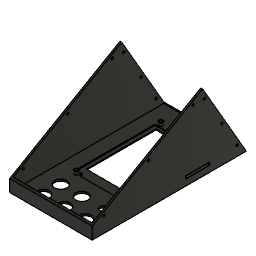
TheShutterTester3_5_screen (Autodesk Fusion 360 design; units mm, degrees)
Autodesk Fusion 360 part; units mm, degrees
sketch "Sketch1" plane through (0, 0, 0) normal (0, 0, 1) x (1, 0, 0)
  line L0 (45, 145.5) -> (45, 50) construction
  line L1 (45, 50) -> (45, 0) construction
  line L2 (0, 14.5) -> (90, 14.5) construction
  line L3 (0, 33.75) -> (90, 33.75) construction
  line L4 (45, 33.75) -> (45, 14.5) construction
  line L5 (22, 33.75) -> (22, 14.5) construction
  line L6 (68, 33.75) -> (68, 14.5) construction
  line L7 (0, 0) -> (90, 0)
  line L8 (90, 0) -> (90, 168)
  line L9 (90, 168) -> (0, 168)
  line L10 (0, 168) -> (0, 0)
  circle A0 centre (45, 33.75) radius 6.7
  circle A1 centre (68, 14.5) radius 6.7
  circle A2 centre (45, 14.5) radius 6.7
  circle A3 centre (22, 14.5) radius 6.7
  circle A4 centre (22, 33.75) radius 6.7
  circle A5 centre (68, 33.75) radius 3.7
  line L11 (13.5, 52) -> (0, 52) construction
  line L12 (13.5, 79) -> (0, 79) construction
  line L13 (73.17, 49) -> (16.83, 49) construction
  line L14 (16.83, 49) -> (16.83, 147) construction
  line L15 (16.83, 147) -> (73.17, 147) construction
  line L16 (73.17, 147) -> (73.17, 49) construction
  circle A6 centre (20.25, 144.5) radius 1.7
  circle A7 centre (69.75, 144.5) radius 1.7
  circle A8 centre (20.25, 52.5) radius 1.7
  circle A9 centre (69.75, 52.5) radius 1.7
  circle A10 centre (20.25, 144.5) radius 2.4
  circle A11 centre (69.75, 52.5) radius 2.4
  line L17 (73.17, 141.0151) -> (72.7211, 141.0151)
  line L18 (73.17, 141.6) -> (16.83, 141.6)
  line L19 (16.83, 141.6) -> (16.83, 55.4)
  line L20 (73.17, 55.4) -> (73.17, 141.6)
  line L21 (20.83, 138.6) -> (20.83, 63)
  line L22 (69.17, 63) -> (69.17, 138.6)
  line L23 (69.17, 138.6) -> (20.83, 138.6)
  circle A12 centre (20.25, 52.5) radius 2.4
  line L24 (66.2226, 55.4) -> (66.2226, 52)
  line L25 (66.2226, 52) -> (57, 52)
  line L26 (66.2226, 55.4) -> (73.17, 55.4)
  line L27 (57, 52) -> (52, 52)
  line L28 (52, 52) -> (24, 52)
  line L29 (24, 52) -> (24, 55.4)
  line L30 (16.83, 55.4) -> (24, 55.4)
  line L31 (45, 55.4) -> (52, 55.4)
  circle A13 centre (69.75, 144.5) radius 2.4
  line L32 (20.83, 63) -> (69.17, 63)
  point P0 (90, 168)
  point P1 (90, 168)
  point P2 (45, 145.5)
  point P3 (45, 0)
  point P4 (17.42, 149)
  point P5 (72.58, 47)
  point P6 (72.58, 149)
  point P7 (22, 33.75)
  point P8 (22, 14.5)
  point P9 (45, 14.5)
  point P10 (45, 33.75)
  point P11 (68, 33.75)
  point P12 (68, 14.5)
  point P13 (0, 158)
  point P14 (90, 0)
  point P15 (110, -10)
  point P16 (17.42, 47)
  point P17 (72.58, 47)
  point P18 (0, 52)
  point P19 (0, 79)
  point P20 (75.5, 98)
  point P21 (45, 97.75)
  point P22 (16.83, 147)
  point P23 (73.17, 49)
  point P24 (69.75, 144.5)
  point P25 (20.25, 144.5)
  point P26 (69.75, 52.5)
  point P27 (20.25, 52.5)
  dimension "d158" = 168
  dimension "d159" = 90
  dimension "d163" = 13.4
  dimension "d165" = 13.4
  dimension "d166" = 13.4
  dimension "d167" = 13.4
  dimension "d190" = 13.4
  dimension "d191" = 7.4
  dimension "d257" = 3.4
  dimension "d258" = 3.4
  dimension "d259" = 3.4
  dimension "d260" = 3.4
  dimension "d261" = 4.8
  dimension "d264" = 4.8
  dimension "d268" = 4.8
  dimension "d280" = 4.8
  constraint coincident P0 L8.end
  constraint coincident P2 L0.start
  constraint coincident P3 L1.end
  constraint horizontal L2
  constraint horizontal L3
  constraint midpoint L3 P10
  constraint midpoint L2 P9
  constraint perpendicular L2 L4
  constraint coincident P7 L5.start
  constraint coincident P8 L5.end
  constraint coincident P9 L4.end
  constraint coincident P10 L4.start
  constraint coincident P11 L6.start
  constraint coincident P12 L6.end
  constraint coincident P17 P5
  constraint horizontal L7
  constraint vertical L8
  constraint horizontal L9
  constraint vertical L10
  constraint coincident P1 P0
  constraint coincident L7.start L10.end
  constraint coincident P18 L11.end
  constraint coincident P19 L12.end
  constraint midpoint L0 P21
  constraint horizontal L13
  constraint vertical L14
  constraint horizontal L15
  constraint vertical L16
  constraint coincident P22 L14.end
  constraint coincident P23 L13.start
  constraint coincident P25 A6.centre
  constraint coincident P24 A7.centre
  constraint coincident P27 A8.centre
  constraint coincident P26 A9.centre
  constraint concentric A9 A11
  constraint coincident L14 L19.end
  constraint coincident L16 L20.start
  constraint perpendicular L16 L26
  constraint coincident L16 L17.start
  constraint perpendicular L16 L17
  constraint coincident L16 L18.start
  constraint coincident L14 L18.end
  constraint perpendicular L14 L18
  constraint perpendicular L13 L24
  constraint perpendicular L24 L25
  constraint collinear L26 L31
  constraint perpendicular L0 L28
  constraint perpendicular L29 L30
  constraint coincident L0 L31.start
  constraint collinear L30 L31
  measures "d158" distance of P14 P1
  measures "d159" distance of P1 L9.end
  measures "d163" diameter of A0
  measures "d165" diameter of A1
  measures "d166" diameter of A2
  measures "d167" diameter of A3
  measures "d190" diameter of A4
  measures "d191" diameter of A5
  measures "d257" diameter of A6
  measures "d258" diameter of A7
  measures "d259" diameter of A8
  measures "d260" diameter of A9
  measures "d261" diameter of A10
  measures "d264" diameter of A11
  measures "d268" diameter of A12
  measures "d280" diameter of A13
extrude "Extrude24" add sketch "Sketch1" along normal blind 2 contours L7 L8 L9 L10
extrude "Extrude21" add sketch "Sketch1" along normal blind 1 contours L18 L19 L20 L24 L25 L26 L27 L28 L29 L30
extrude "Extrude30" add sketch "Sketch1" along normal blind 5 contours A10 | A11 | A12 | A13
sketch "Sketch40" plane through (0, 0, 2) normal (0, 0, 1) x (-1, 0, 0)
  circle A0 centre (-20.25, -52.5) radius 2.4
  circle A1 centre (-20.25, -144.5) radius 2.4
  circle A2 centre (-69.75, -52.5) radius 2.4
  circle A3 centre (-22, -33.75) radius 6.7
  circle A4 centre (-22, -14.5) radius 6.7
  circle A5 centre (-45, -33.75) radius 6.7
  circle A6 centre (-68, -14.5) radius 6.7
  circle A7 centre (-68, -33.75) radius 3.7
  circle A8 centre (-45, -14.5) radius 6.7
  line L0 (0, -168) -> (0, 0)
  line L1 (0, 0) -> (-90, 0)
  line L2 (-90, 0) -> (-90, -168)
  line L3 (-90, -168) -> (0, -168)
  line L4 (0, 0) -> (-90, 0)
  line L5 (0, -168) -> (0, 0)
  line L6 (-90, 0) -> (-90, -168)
  line L7 (-90, -168) -> (0, -168)
  line L8 (-2, -2) -> (-88, -2)
  line L9 (-88, -2) -> (-88, -166)
  line L10 (-88, -166) -> (-2, -166)
  line L11 (-2, -166) -> (-2, -2)
  circle A9 centre (-69.75, -144.5) radius 2.4
  line L12 (-73.17, -55.4) -> (-66.2226, -55.4)
  line L13 (-66.2226, -55.4) -> (-66.2226, -52)
  line L14 (-66.2226, -52) -> (-24, -52)
  line L15 (-24, -52) -> (-24, -55.4)
  line L16 (-24, -55.4) -> (-16.83, -55.4)
  line L17 (-16.83, -55.4) -> (-16.83, -141.6)
  line L18 (-16.83, -141.6) -> (-73.17, -141.6)
  line L19 (-73.17, -141.6) -> (-73.17, -55.4)
  dimension "d279" = -2
extrude "Extrude22" add sketch "Sketch40" along normal blind 150 contours L0 L1 L2 L3 L4 L5 L6 L7
sketch "Sketch29" plane through (90, 0, 0) normal (1, 0, 0) x (0, 1, 0)
  line L0 (168, 0) -> (168, 152)
  line L1 (168, 152) -> (0, 152)
  line L2 (0, 152) -> (0, 0)
  line L3 (0, 13.2763) -> (280.5086, 13.2763) construction
  line L4 (168, 0) -> (120.2512, 82.7033)
  line L5 (0, 13.2763) -> (120.2512, 82.7033)
  line L6 (0, 0) -> (168, 0)
  point P0 (0, 13.2763)
  constraint horizontal L3
  constraint coincident L3 P0
  constraint coincident L2 P0
  constraint coincident P0 L5
  constraint coincident L0.start L4.start
  constraint perpendicular L4 L5
extrude "Extrude23" cut sketch "Sketch29" against normal blind 90 contours L0 L1 L2 L4 L5
sketch "Sketch20" plane through (0, 0, 0) normal (0, 0, 1) x (1, 0, 0)
form "Form1" [no effect]
sketch "Sketch34" plane through (0, 126, 72.7461) normal (0, 0.866025, 0.5) x (-1, 0, 0)
  line L0 (-88, 11.4976) -> (-90, 11.4976)
  line L1 (-90, 11.4976) -> (-90, -84)
  line L2 (0, -84) -> (0, 11.4976)
  line L3 (-90, -84) -> (0, -84)
  line L4 (-88, -80) -> (-88, 11.4976)
  line L5 (0, 11.4976) -> (-2, 11.4976)
  line L6 (-2, 11.4976) -> (-2, -80)
  line L7 (-2, -80) -> (-88, -80)
sketch "Sketch38" plane through (88, 0, 0) normal (-1, 0, 0) x (0, -1, 0)
  circle A0 centre (-61.5586, 44.1983) radius 1.25
  circle A1 centre (-12.9904, 16.1575) radius 1.25
  circle A2 centre (-110.1269, 72.2392) radius 1.25
  circle A3 centre (-141.7043, 39.5456) radius 1.25
  circle A4 centre (-122.7043, 72.4545) radius 1.25
  circle A5 centre (-158.2043, 10.9667) radius 1.25
  line L0 (-120.2512, 82.7033) -> (-166, 3.4641)
  line L1 (-166, 3.4641) -> (-166, 2)
  line L2 (-166, 2) -> (-2, 2)
  line L3 (-2, 2) -> (-2, 14.431)
  line L4 (-2, 14.431) -> (-120.2512, 82.7033)
  line L5 (-128, 6.8) -> (-102, 6.8)
  line L6 (-128, 9.8) -> (-102, 9.8)
  line L7 (-128, 9.8) -> (-128, 6.8)
  line L8 (-102, 9.8) -> (-102, 6.8)
  line L9 (-131, 0) -> (-131, 6.8)
  line L10 (-99, 0) -> (-99, 6.8)
  line L11 (-99, 9.8) -> (-99, 6.8)
  line L12 (-131, 6.8) -> (-131, 13)
  line L13 (-99, 9.8) -> (-99, 13)
  line L14 (-131, 13) -> (-99, 13)
  line L15 (-120.2512, 82.7033) -> (0, 13.2763)
  line L16 (0, 13.2763) -> (0, 0)
  line L17 (0, 0) -> (-168, 0)
  line L18 (-168, 0) -> (-120.2512, 82.7033)
  line L19 (-120.2512, 82.7033) -> (-166, 3.4641)
  line L20 (-166, 3.4641) -> (-166, 2)
  line L21 (-166, 2) -> (-2, 2)
  line L22 (-2, 2) -> (-2, 14.431)
  line L23 (-2, 14.431) -> (-120.2512, 82.7033)
  constraint perpendicular L5 L7
  constraint perpendicular L5 L8
  constraint parallel L9 L12
  constraint perpendicular L5 L13
  constraint perpendicular L13 L14
extrude "Extrude31" cut sketch "Sketch38" against normal blind 2 contours L5 L6 L7 L8
extrude "Extrude32" add sketch "Sketch38" along normal blind 14 contours L2 L9 L10 L11 L12 L13 L14 L21
sketch "Sketch41" plane through (90, 0, 0) normal (1, 0, 0) x (0, 1, 0)
  line L0 (128, 6.8) -> (102, 6.8)
  line L1 (102, 6.8) -> (102, 9.8)
  line L2 (102, 9.8) -> (128, 9.8)
  line L3 (128, 9.8) -> (128, 6.8)
  line L4 (120.2512, 82.7033) -> (0, 13.2763)
  line L5 (0, 13.2763) -> (0, 0)
  line L6 (0, 0) -> (168, 0)
  line L7 (168, 0) -> (120.2512, 82.7033)
  line L8 (168, 0) -> (120.2512, 82.7033)
  line L9 (120.2512, 82.7033) -> (0, 13.2763)
  line L10 (0, 0) -> (168, 0)
  line L11 (164, 0) -> (117.2512, 80.9713) construction
  line L12 (120.2512, 82.7033) -> (0, 13.2763)
  line L13 (120.2512, 82.7033) -> (0, 13.2763)
  line L14 (120.2512, 78.7033) -> (0, 9.2763) construction
  line L15 (120.2512, 78.7033) -> (121.9833, 79.7033) construction
  point P0 (117.2512, 80.9713)
  point P1 (122.2512, 72.311)
  point P2 (141.2512, 39.4021)
  point P3 (157.7512, 10.8232)
  point P4 (109.8589, 72.7033)
  point P5 (61.3615, 44.7033)
  point P6 (12.8641, 16.7033)
  point P7 (12.8641, 16.7033)
  dimension "d281" = 10
  dimension "d282" = 48
  dimension "d283" = 81
  dimension "d284" = 14
  dimension "d285" = 70
  dimension "d286" = 126
  constraint coincident L4 P0
  constraint coincident P0 L11.end
  constraint coincident L8 L15.end
  constraint perpendicular L8 L15
  measures "d281" distance of P0 P1
  measures "d282" distance of P0 P2
  measures "d283" distance of P0 P3
  measures "d284" distance of L15.end P4
  measures "d285" distance of L15.end P5
  measures "d286" distance of L15.end P7
hole "Hole14" at (90, 12.8641, 16.7033) at (90, 61.3615, 44.7033) at (90, 109.8589, 72.7033) at (90, 122.2512, 72.311) at (90, 141.2512, 39.4021) at (90, 157.7512, 10.8232) direction (-1, 0, 0) diameter 2.5 depth 90 tip angle 180
